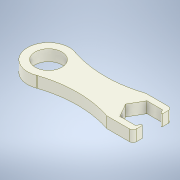
# Autodesk Inventor part: ShortLink
Saved by Autodesk Inventor 2022 (Build 260153000, 153)
## iProperties
Created: 2021-12-08
Part Number: ShortLink
Material: Genérico
Document SubType Name: Modeling
Designer: JK
Density: 1 g/cm^3
Appearance: Suave - Marfil
Author: JK
Autodesk Inventor part; units mm, degrees
ref_plane "YZ Plane" through (0, 0, 0) normal (1, 0, 0) x (0, 1, 0)
ref_plane "XZ Plane" through (0, 0, 0) normal (0, 1, 0) x (-1, 0, 0)
ref_plane "XY Plane" through (0, 0, 0) normal (0, 0, 1) x (1, 0, 0)
sketch "Boceto1" plane through (0, 0, 0) normal (0, 1, 0) x (-1, 0, 0)
  line L0 (6.0622, 0) -> (3.0311, -5.25)
  line L1 (3.0311, -5.25) -> (-3.0311, -5.25)
  line L2 (-3.0311, -5.25) -> (-6.0622, 0)
  line L3 (-6.0622, 0) -> (-3.0311, 5.25)
  line L4 (-3.0311, 5.25) -> (3.0311, 5.25)
  line L5 (3.0311, 5.25) -> (6.0622, 0)
  circle A0 centre (0, 0) radius 5.25
  line L6 (4.2147, 0) -> (2.1073, -3.65)
  line L7 (2.1073, -3.65) -> (-2.1073, -3.65)
  line L8 (-2.1073, -3.65) -> (-4.2147, 0)
  line L9 (-4.2147, 0) -> (-2.1073, 3.65)
  line L10 (-2.1073, 3.65) -> (2.1073, 3.65)
  line L11 (2.1073, 3.65) -> (4.2147, 0)
  dimension "d0" = 10.5
  dimension "d4" = 1.6
  constraints: 24 end point, 2 coincident, 1 centre point, 1 tangent, 18 other
  measures "d0" diameter of A0
  measures "d4" distance between parallel lines of L2 L8
extrude "Extrusión1" add sketch "Boceto1" along normal blind 3
sketch "Boceto2" plane through (0, 3, 0) normal (0, 1, 0) x (1, 0, 0)
  line L0 (5.3982, 6.1665) -> (3.0311, 6.1665)
  line L1 (3.0311, 6.1665) -> (3.0311, -6.1665)
  line L2 (3.0311, -6.1665) -> (5.3982, -6.1665)
  line L3 (5.3982, -6.1665) -> (5.3982, 6.1665)
  line L4 (2.1073, 3.65) -> (4.2147, 0) projected
  line L5 (5.3982, 6.1665) -> (3.0311, -6.1665) construction
  line L6 (3.0311, 6.1665) -> (5.3982, -6.1665) construction
  line L7 (3.0311, -5.25) -> (6.0622, 0) projected
  circle A0 centre (6.0622, 0) radius 2.2925
  point P0 (0, 0)
  point P1 (5.3982, 2.1942)
  point P2 (5.3982, -2.1942)
  constraints: 12 end point, 2 midpoint, 2 parallel, 1 centre point, 1 horizontal, 1 perpendicular, 1 point on line
extrude "Extrusión2" cut sketch "Boceto2" against normal blind 3
fillet "Empalme1" radius 1 4 edges at (3.0311, 1.5, -5.25) (3.0311, 1.5, 5.25) (-3.0311, 1.5, 5.25) (-3.0311, 1.5, -5.25)
fillet "Empalme2" radius 0.2 2 edges at (3.0311, 1.5, -2.05) (3.0311, 1.5, 2.05)
sketch "Boceto3" plane through (0, 3, 0) normal (0, 1, 0) x (1, 0, 0)
  line L0 (-22.9119, 5.25) -> (-4.2147, 5.25)
  line L1 (-4.2147, 5.25) -> (-4.2147, -5.25)
  line L2 (-4.2147, -5.25) -> (-22.9119, -5.25)
  line L3 (-22.9119, -5.25) -> (-22.9119, 5.25)
  line L4 (-22.9119, 5.25) -> (-4.2147, -5.25) construction
  line L5 (-4.2147, 5.25) -> (-22.9119, -5.25) construction
  line L6 (2.6579, -2.6964) -> (2.1073, -3.65) projected
  line L7 (2.1073, -3.65) -> (-2.1073, -3.65) projected
  line L8 (-2.1073, -3.65) -> (-4.2147, 0) projected
  line L9 (-4.2147, 0) -> (-2.1073, 3.65) projected
  line L10 (-2.1073, 3.65) -> (2.1073, 3.65) projected
  line L11 (2.1073, 3.65) -> (2.6579, 2.6964) projected
  arc A0 (3.0311, 4.25) -> (2.0311, 5.25) centre (2.0311, 4.25) ccw projected
  line L12 (2.0311, 5.25) -> (-2.4537, 5.25) projected
  arc A1 (-2.4537, 5.25) -> (-3.3198, 4.75) centre (-2.4537, 4.25) ccw projected
  line L13 (-3.3198, 4.75) -> (-6.0622, 0) projected
  line L14 (-6.0622, 0) -> (-3.3198, -4.75) projected
  arc A2 (-3.3198, -4.75) -> (-2.4537, -5.25) centre (-2.4537, -4.25) ccw projected
  line L15 (-2.4537, -5.25) -> (2.0311, -5.25) projected
  arc A3 (2.0311, -5.25) -> (3.0311, -4.25) centre (2.0311, -4.25) ccw projected
  line L16 (-4.2147, 5.25) -> (-0.7217, 5.25)
  line L17 (-0.7217, 5.25) -> (-0.7217, -5.25)
  line L18 (-0.7217, -5.25) -> (-4.2147, -5.25)
  line L19 (-4.2147, -5.25) -> (-4.2147, 5.25)
  circle A4 centre (-25, 0) radius 3.6
  circle A5 centre (-25, 0) radius 5.65
  arc A6 (3.0311, -2.7964) -> (2.6579, -2.6964) centre (2.8311, -2.7964) ccw projected
  arc A7 (2.6579, 2.6964) -> (3.0311, 2.7964) centre (2.8311, 2.7964) ccw projected
  line L20 (3.0311, 2.7964) -> (3.0311, 4.25) projected
  line L21 (3.0311, -4.25) -> (3.0311, -2.7964) projected
  point P0 (0, 0)
  point P1 (-13.5633, 0)
  point P2 (-13.5633, 0)
  point P3 (-13.5633, 0)
  point P4 (-2.4537, -5.25)
  point P5 (-2.4537, 5.25)
  point P6 (-22.9119, 5.25)
  point P7 (-2.8868, 4)
  point P8 (-4.2147, 3.2)
  point P9 (-4.2147, -3.2)
  point P10 (-22.9119, 5.25)
  point P11 (-0.7217, -3.65)
  point P12 (-0.7217, 3.65)
  point P13 (-0.7217, 5.25)
  dimension "d12" = 11.3
  dimension "d10" = 25
  dimension "d11" = 7.2
  constraints: 20 end point, 5 midpoint, 4 parallel, 2 horizontal, 2 horizontal alignment, 2 perpendicular, 1 centre point, 1 coincident, 1 collinear, 1 point on line, 3 other
  measures "d10" distance of point (0, 0) A4.centre
  measures "d11" diameter of A4
extrude "Extrusión3" add sketch "Boceto3" against normal up to surface (3 mm away) contours A5 L3 A4 | L0 L1 L13 L14 L2 A5 | L3 A4 A5 | L16 A1 L13 L1 | L1 L14 A2 L18
sketch "Boceto4" plane through (0, 3, 0) normal (0, 1, 0) x (1, 0, 0)
  line L0 (2.0311, 5.25) -> (-22.9119, 5.25) projected
  arc A0 (-22.9119, 5.25) -> (-4, 5.25) centre (-13.456, 33.7208) ccw
  line L1 (-22.9119, -5.25) -> (2.0311, -5.25) projected
  arc A1 (-4, -5.25) -> (-22.9119, -5.25) centre (-13.456, -33.7208) ccw
  circle A2 centre (-25, 0) radius 3.6 projected
  arc A3 (3.0311, -2.7964) -> (2.6579, -2.6964) centre (2.8311, -2.7964) ccw projected
  line L2 (2.6579, -2.6964) -> (2.1073, -3.65) projected
  line L3 (2.1073, -3.65) -> (-2.1073, -3.65) projected
  line L4 (-2.1073, -3.65) -> (-4.2147, 0) projected
  line L5 (-4.2147, 0) -> (-2.1073, 3.65) projected
  line L6 (-2.1073, 3.65) -> (2.1073, 3.65) projected
  line L7 (2.1073, 3.65) -> (2.6579, 2.6964) projected
  arc A4 (2.6579, 2.6964) -> (3.0311, 2.7964) centre (2.8311, 2.7964) ccw projected
  line L8 (3.0311, 2.7964) -> (3.0311, 4.25) projected
  arc A5 (3.0311, 4.25) -> (2.0311, 5.25) centre (2.0311, 4.25) ccw projected
  line L9 (2.0311, 5.25) -> (-22.9119, 5.25) projected
  arc A6 (-22.9119, 5.25) -> (-22.9119, -5.25) centre (-25, 0) ccw projected
  line L10 (-22.9119, -5.25) -> (2.0311, -5.25) projected
  arc A7 (2.0311, -5.25) -> (3.0311, -4.25) centre (2.0311, -4.25) ccw projected
  line L11 (3.0311, -4.25) -> (3.0311, -2.7964) projected
  point P0 (0, 0)
  dimension "d16" = 4
  dimension "d18" = 30
  constraints: 4 point on circle, 2 centre point, 2 point on line, 1 equal radius, 1 vertical alignment
  measures "d16" horizontal distance of point (0, 0) A0.end
  measures "d18" radius of A0
extrude "Extrusión4" cut sketch "Boceto4" against normal through all contours A0 L0 | A1 L1
fillet "Empalme4" radius 3 2 edges at (-22.9119, 1.5, -5.25) (-22.9119, 1.5, 5.25)
